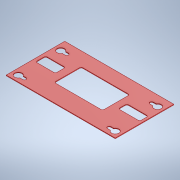
# Autodesk Inventor part: Cockpit_back_frame_cloth
Saved by Autodesk Inventor 2022 (Build 260153000, 153)
## iProperties
Part Number: Cockpit_back_frame_cloth
Material: PET プラスチック
Document SubType Name: Modeling
Designer: Masato Kubotera
Density: 1.541 g/cm^3
Appearance: 滑らか - 赤
Description: PP T0.75
Mass: 7.54732 g
Surface Area: 137.43 cm^2
Volume: 4.89767 cm^3
Author: Masato Kubotera
Autodesk Inventor part; units mm, degrees
ref_plane "YZ Plane" through (0, 0, 0) normal (1, 0, 0) x (0, 1, 0)
ref_plane "XZ Plane" through (0, 0, 0) normal (0, 1, 0) x (-1, 0, 0)
derived "Cockpit_back_frame.ipt"
sketch "スケッチ3" plane through (-88.25, 0, 0) normal (1, 0, 0) x (0, 1, 0)
  line L0 (-135, -22.5) -> (0, -22.5)
  line L1 (0, -22.5) -> (0, -39.7651)
  line L2 (0, -90) -> (-135, -90)
  line L3 (-135, -56.25) -> (0, -56.25) construction
  line L4 (-67.5, -22.5) -> (-67.5, -90) construction
  line L5 (1.4849, -41.25) -> (5, -41.25)
  line L6 (5, -41.25) -> (5, -71.25)
  line L7 (5, -71.25) -> (1.4849, -71.25)
  arc A0 (0, -39.7651) -> (1.4849, -41.25) centre (0.7425, -40.5075) ccw
  arc A1 (1.4849, -71.25) -> (0, -72.7349) centre (0.7425, -71.9925) ccw
  line L8 (0, -41.25) -> (0, -71.25)
  line L9 (0, -72.7349) -> (0, -90)
  line L10 (-135, -41.25) -> (-135, -71.25)
  line L11 (-135, -22.5) -> (-135, -39.7651)
  arc A2 (-136.4849, -41.25) -> (-135, -39.7651) centre (-135.7425, -40.5075) ccw
  line L12 (-136.4849, -41.25) -> (-140, -41.25)
  line L13 (-140, -41.25) -> (-140, -71.25)
  line L14 (-135, -72.7349) -> (-135, -90)
  arc A3 (-135, -72.7349) -> (-136.4849, -71.25) centre (-135.7425, -71.9925) ccw
  line L15 (-140, -71.25) -> (-136.4849, -71.25)
  line L16 (-100.5, -34.65) -> (-34.5, -34.65)
  line L17 (-32.5, -36.65) -> (-32.5, -66.15)
  line L18 (-34.5, -68.15) -> (-100.5, -68.15)
  line L19 (-102.5, -66.15) -> (-102.5, -36.65)
  arc A4 (-100.5, -34.65) -> (-102.5, -36.65) centre (-100.5, -36.65) ccw
  arc A5 (-102.5, -66.15) -> (-100.5, -68.15) centre (-100.5, -66.15) ccw
  arc A6 (-34.5, -68.15) -> (-32.5, -66.15) centre (-34.5, -66.15) ccw
  arc A7 (-32.5, -36.65) -> (-34.5, -34.65) centre (-34.5, -36.65) ccw
  line L20 (-126.5, -47.35) -> (-126.5, -55.45) construction
  line L21 (-118.75, -47.1) -> (-118.75, -55.7) construction
  line L22 (-110.75, -47.1) -> (-126.75, -47.1)
  line L23 (-126.75, -55.7) -> (-110.75, -47.1) construction
  line L24 (-110.75, -55.7) -> (-126.75, -47.1) construction
  line L25 (-111, -47.35) -> (-126.5, -47.35) construction
  line L26 (-111, -55.45) -> (-111, -47.35) construction
  line L27 (-111, -47.35) -> (-126.5, -55.45) construction
  circle A8 centre (-108.75, -51.4) radius 1.35
  circle A9 centre (-108.75, -51.4) radius 2.25 construction
  line L28 (-126.5, -47.35) -> (-111, -55.45) construction
  circle A10 centre (-128.75, -51.4) radius 1.35
  line L29 (-110.75, -55.7) -> (-110.75, -47.1)
  line L30 (-126.75, -55.7) -> (-110.75, -55.7)
  line L31 (-126.5, -55.45) -> (-111, -55.45) construction
  line L32 (-108.75, -51.4) -> (-128.75, -51.4) construction
  line L33 (-126.75, -47.1) -> (-126.75, -55.7)
  line L34 (-27.5, -56.65) -> (-5, -56.65) construction
  line L35 (-16.25, -46.15) -> (-16.25, -56.65) construction
  line L36 (-5, -46.15) -> (-27.5, -46.15) construction
  line L37 (-27.5, -46.15) -> (-5, -56.65) construction
  line L38 (-27.5, -56.65) -> (-5, -46.15) construction
  line L39 (-27.75, -56.9) -> (-4.75, -56.9)
  line L40 (-4.75, -45.9) -> (-27.75, -45.9)
  line L41 (-27.75, -45.9) -> (-4.75, -56.9) construction
  line L42 (-27.75, -56.9) -> (-4.75, -45.9) construction
  line L43 (-29.25, -51.4) -> (-3.25, -51.4) construction
  arc A11 (-6.2349, -56.9) -> (-4.75, -55.4151) centre (-5.4925, -56.1575) ccw
  line L44 (-5, -56.65) -> (-5, -46.15) construction
  line L45 (-4.75, -56.9) -> (-4.75, -45.9)
  arc A12 (-4.75, -47.3849) -> (-6.2349, -45.9) centre (-5.4925, -46.6425) ccw
  circle A13 centre (-3.25, -51.4) radius 0.8
  line L46 (-27.5, -46.15) -> (-27.5, -56.65) construction
  line L47 (-27.75, -45.9) -> (-27.75, -56.9)
  arc A14 (-26.2651, -45.9) -> (-27.75, -47.3849) centre (-27.0075, -46.6425) ccw
  arc A15 (-27.75, -55.4151) -> (-26.2651, -56.9) centre (-27.0075, -56.1575) ccw
  circle A16 centre (-29.25, -51.4) radius 0.8
  arc A17 (-110.75, -48.5849) -> (-112.2349, -47.1) centre (-111.4925, -47.8425) ccw
  arc A18 (-112.2349, -55.7) -> (-110.75, -54.2151) centre (-111.4925, -54.9575) ccw
  arc A19 (-126.75, -54.2151) -> (-125.2651, -55.7) centre (-126.0075, -54.9575) ccw
  arc A20 (-125.2651, -47.1) -> (-126.75, -48.5849) centre (-126.0075, -47.8425) ccw
  line L48 (-130, -29.5) -> (-130, -41.65)
  line L49 (-128, -43.65) -> (-107, -43.65)
  line L50 (-128, -27.5) -> (-126, -27.5)
  line L51 (-105, -29.5) -> (-105, -41.65)
  line L52 (-28, -27.5) -> (-21, -27.5)
  line L53 (-5, -29.5) -> (-5, -41.65)
  line L54 (-7, -43.65) -> (-28, -43.65)
  line L55 (-30, -41.65) -> (-30, -29.5)
  line L56 (-100.5, -27.5) -> (-34.5, -27.5)
  line L57 (-32.5, -29.5) -> (-32.5, -30.15)
  line L58 (-34.5, -32.15) -> (-100.5, -32.15)
  line L59 (-102.5, -30.15) -> (-102.5, -29.5)
  line L60 (-128, -59.15) -> (-107, -59.15)
  line L61 (-7, -59.15) -> (-28, -59.15)
  line L62 (-34.5, -70.65) -> (-100.5, -70.65)
  line L63 (-100.5, -85) -> (-34.5, -85)
  line L64 (-128, -85) -> (-126, -85)
  line L65 (-28, -85) -> (-21, -85)
  line L66 (-130, -61.15) -> (-130, -83)
  line L67 (-105, -61.15) -> (-105, -83)
  line L68 (-102.5, -83) -> (-102.5, -72.65)
  line L69 (-32.5, -72.65) -> (-32.5, -83)
  line L70 (-30, -83) -> (-30, -61.15)
  line L71 (-5, -61.15) -> (-5, -83)
  arc A21 (-128, -27.5) -> (-130, -29.5) centre (-128, -29.5) ccw
  arc A22 (-130, -41.65) -> (-128, -43.65) centre (-128, -41.65) ccw
  arc A23 (-107, -43.65) -> (-105, -41.65) centre (-107, -41.65) ccw
  arc A24 (-105, -29.5) -> (-107, -27.5) centre (-107, -29.5) ccw
  arc A25 (-100.5, -27.5) -> (-102.5, -29.5) centre (-100.5, -29.5) ccw
  arc A26 (-102.5, -30.15) -> (-100.5, -32.15) centre (-100.5, -30.15) ccw
  arc A27 (-34.5, -32.15) -> (-32.5, -30.15) centre (-34.5, -30.15) ccw
  arc A28 (-32.5, -29.5) -> (-34.5, -27.5) centre (-34.5, -29.5) ccw
  arc A29 (-28, -27.5) -> (-30, -29.5) centre (-28, -29.5) ccw
  arc A30 (-5, -29.5) -> (-7, -27.5) centre (-7, -29.5) ccw
  arc A31 (-7, -43.65) -> (-5, -41.65) centre (-7, -41.65) ccw
  arc A32 (-30, -41.65) -> (-28, -43.65) centre (-28, -41.65) ccw
  arc A33 (-28, -59.15) -> (-30, -61.15) centre (-28, -61.15) ccw
  arc A34 (-30, -83) -> (-28, -85) centre (-28, -83) ccw
  arc A35 (-7, -85) -> (-5, -83) centre (-7, -83) ccw
  arc A36 (-5, -61.15) -> (-7, -59.15) centre (-7, -61.15) ccw
  arc A37 (-34.5, -85) -> (-32.5, -83) centre (-34.5, -83) ccw
  arc A38 (-32.5, -72.65) -> (-34.5, -70.65) centre (-34.5, -72.65) ccw
  arc A39 (-102.5, -83) -> (-100.5, -85) centre (-100.5, -83) ccw
  arc A40 (-100.5, -70.65) -> (-102.5, -72.65) centre (-100.5, -72.65) ccw
  arc A41 (-107, -85) -> (-105, -83) centre (-107, -83) ccw
  arc A42 (-105, -61.15) -> (-107, -59.15) centre (-107, -61.15) ccw
  arc A43 (-128, -59.15) -> (-130, -61.15) centre (-128, -61.15) ccw
  arc A44 (-130, -83) -> (-128, -85) centre (-128, -83) ccw
  arc A45 (-15, -27.9) -> (-15, -32.1) centre (-15, -30) ccw construction
  circle A46 centre (-15, -30) radius 2
  circle A47 centre (-15, -30) radius 3 construction
  line L72 (-15, -32.1) -> (-11.4799, -32.1) construction
  line L73 (-15, -27.9) -> (-11.4799, -27.9) construction
  line L74 (-7.5, -30) -> (-15, -30) construction
  arc A48 (-11.4799, -32.1) -> (-11.4799, -27.9) centre (-7.5, -30) ccw construction
  arc A49 (-19, -30) -> (-11, -30) centre (-15, -30) ccw
  line L75 (-11, -30) -> (-11, -29.5)
  line L76 (-19, -30) -> (-19, -29.5)
  line L77 (-9, -27.5) -> (-7, -27.5)
  line L78 (-116, -30) -> (-116, -29.5)
  arc A50 (-124, -30) -> (-116, -30) centre (-120, -30) ccw
  circle A51 centre (-120, -30) radius 3 construction
  line L79 (-120, -32.1) -> (-123.5201, -32.1) construction
  line L80 (-120, -27.9) -> (-123.5201, -27.9) construction
  arc A52 (-120, -32.1) -> (-120, -27.9) centre (-120, -30) ccw construction
  circle A53 centre (-120, -30) radius 2
  arc A54 (-123.5201, -27.9) -> (-123.5201, -32.1) centre (-127.5, -30) ccw construction
  line L81 (-124, -30) -> (-124, -29.5)
  line L82 (-114, -27.5) -> (-107, -27.5)
  arc A55 (-123.5201, -80.4) -> (-123.5201, -84.6) centre (-127.5, -82.5) ccw construction
  line L83 (-120, -84.6) -> (-123.5201, -84.6) construction
  circle A56 centre (-120, -82.5) radius 3 construction
  circle A57 centre (-120, -82.5) radius 2
  arc A58 (-120, -84.6) -> (-120, -80.4) centre (-120, -82.5) ccw construction
  line L84 (-124, -82.5) -> (-124, -83)
  arc A59 (-116, -82.5) -> (-124, -82.5) centre (-120, -82.5) ccw
  line L85 (-116, -82.5) -> (-116, -83)
  arc A60 (-11.4799, -84.6) -> (-11.4799, -80.4) centre (-7.5, -82.5) ccw construction
  line L86 (-15, -84.6) -> (-11.4799, -84.6) construction
  circle A61 centre (-15, -82.5) radius 3 construction
  circle A62 centre (-15, -82.5) radius 2
  arc A63 (-15, -80.4) -> (-15, -84.6) centre (-15, -82.5) ccw construction
  line L87 (-15, -80.4) -> (-11.4799, -80.4) construction
  arc A64 (-11, -82.5) -> (-19, -82.5) centre (-15, -82.5) ccw
  line L88 (-19, -82.5) -> (-19, -83)
  line L89 (-7.5, -82.5) -> (-15, -82.5) construction
  line L90 (-11, -82.5) -> (-11, -83)
  line L91 (-9, -85) -> (-7, -85)
  line L92 (-120, -80.4) -> (-123.5201, -80.4) construction
  line L93 (-114, -85) -> (-107, -85)
  arc A65 (-126, -85) -> (-124, -83) centre (-126, -83) ccw
  arc A66 (-116, -83) -> (-114, -85) centre (-114, -83) ccw
  arc A67 (-124, -29.5) -> (-126, -27.5) centre (-126, -29.5) ccw
  arc A68 (-114, -27.5) -> (-116, -29.5) centre (-114, -29.5) ccw
  arc A69 (-19, -29.5) -> (-21, -27.5) centre (-21, -29.5) ccw
  arc A70 (-9, -27.5) -> (-11, -29.5) centre (-9, -29.5) ccw
  arc A71 (-21, -85) -> (-19, -83) centre (-21, -83) ccw
  arc A72 (-11, -83) -> (-9, -85) centre (-9, -83) ccw
  point P0 (0, 0)
  point P1 (-135, -71.5)
  point P2 (0, -71.5)
  point P3 (-67.5, -34.65)
  point P4 (-118.75, -51.4)
  point P5 (-118.75, -51.4)
  point P6 (-16.25, -51.4)
  point P7 (-16.25, -51.4)
  point P8 (-125, -54.6849)
  point P9 (-123.5151, -53.2)
  point P10 (-110, -60.3151)
  point P11 (-111.4849, -61.8)
  point P12 (-123.5151, -61.8)
  point P13 (-125, -60.3151)
  point P14 (-27.5151, -63)
  point P15 (-29, -61.5151)
  point P16 (-7.4849, -52)
  point P17 (-6, -53.4849)
  point P18 (-6, -61.5151)
  point P19 (-7.4849, -63)
  point P20 (-130, -27.5)
  point P21 (-130, -43.65)
  point P22 (-105, -27.5)
  point P23 (-105, -43.65)
  point P24 (-30, -27.5)
  point P25 (-5, -43.65)
  point P26 (-5, -27.5)
  point P27 (-30, -43.65)
  point P28 (-102.5, -27.5)
  point P29 (-32.5, -32.15)
  point P30 (-32.5, -27.5)
  point P31 (-102.5, -32.15)
  point P32 (-130, -59.15)
  point P33 (-105, -59.15)
  point P34 (-5, -59.15)
  point P35 (-30, -59.15)
  point P36 (-32.5, -70.65)
  point P37 (-102.5, -70.65)
  point P38 (-102.5, -85)
  point P39 (-32.5, -85)
  point P40 (-130, -85)
  point P41 (-105, -85)
  point P42 (-30, -85)
  point P43 (-5, -85)
  point P44 (-135, -71.5)
  point P45 (0, -71.5)
  point P46 (-125.5, -54.6849)
  point P47 (-124.0151, -53.2)
  point P48 (-109.5, -60.3151)
  point P49 (-110.9849, -61.8)
  point P50 (-124.0151, -61.8)
  point P51 (-125.5, -60.3151)
  point P52 (-27.5151, -63)
  point P53 (-29, -61.5151)
  point P54 (-7.4849, -52)
  point P55 (-6, -53.4849)
  point P56 (-6, -61.5151)
  point P57 (-7.4849, -63)
  point P58 (-102.5, -51.4)
  point P59 (-11, -27.5)
  point P60 (-19, -27.5)
  point P61 (-3, -30)
  point P62 (-116, -27.5)
  point P63 (-124, -27.5)
  point P64 (-124, -85)
  point P65 (-116, -85)
  point P66 (-19, -85)
  point P67 (-11, -85)
  point P68 (-118.75, -43.65)
  point P69 (-118.75, -51.4)
  point P70 (-16.25, -51.4)
ref_plane "作業平面1" through (-88.25, -135, -22.5) normal (-1, 0, 0) x (0, 1, 0)
sketch "スケッチ4" plane through (-88.25, -135, -22.5) normal (-1, 0, 0) x (0, 1, 0)
  line L0 (135, 111) -> (135, -2.5) construction
  arc A0 (102.5, 43.65) -> (100.5, 45.65) centre (100.5, 43.65) ccw projected
  line L1 (102.5, 14.15) -> (102.5, 43.65) projected
  arc A1 (100.5, 12.15) -> (102.5, 14.15) centre (100.5, 14.15) ccw projected
  line L2 (34.5, 12.15) -> (100.5, 12.15) projected
  line L3 (100.5, 45.65) -> (34.5, 45.65) projected
  line L4 (32.5, 43.65) -> (32.5, 14.15) projected
  arc A2 (32.5, 14.15) -> (34.5, 12.15) centre (34.5, 14.15) ccw projected
  arc A3 (34.5, 45.65) -> (32.5, 43.65) centre (34.5, 43.65) ccw projected
  line L5 (27.5, 34.2) -> (5, 34.2)
  line L6 (3, 32.2) -> (3, 25.6)
  line L7 (5, 23.6) -> (27.5, 23.6)
  line L8 (29.5, 25.6) -> (29.5, 32.2)
  line L9 (29.5, 34.2) -> (3, 23.6) construction
  line L10 (3, 34.2) -> (29.5, 23.6) construction
  circle A4 centre (26.25, 28.9) radius 2.25 construction
  arc A5 (29.5, 32.2) -> (27.5, 34.2) centre (27.5, 32.2) ccw
  arc A6 (5, 34.2) -> (3, 32.2) centre (5, 32.2) ccw
  arc A7 (3, 25.6) -> (5, 23.6) centre (5, 25.6) ccw
  arc A8 (27.5, 23.6) -> (29.5, 25.6) centre (27.5, 25.6) ccw
  line L11 (130, 34.15) -> (130, 23.65) construction
  line L12 (107.5, 34.15) -> (130, 34.15) construction
  line L13 (108.5, 22.65) -> (129, 22.65)
  line L14 (131, 24.65) -> (131, 33.15)
  line L15 (129, 35.15) -> (108.5, 35.15)
  line L16 (106.5, 33.15) -> (106.5, 24.65)
  line L17 (106.5, 22.65) -> (131, 35.15) construction
  line L18 (131, 22.65) -> (106.5, 35.15) construction
  arc A9 (131, 33.15) -> (129, 35.15) centre (129, 33.15) ccw
  arc A10 (108.5, 35.15) -> (106.5, 33.15) centre (108.5, 33.15) ccw
  arc A11 (106.5, 24.65) -> (108.5, 22.65) centre (108.5, 24.65) ccw
  arc A12 (129, 22.65) -> (131, 24.65) centre (129, 24.65) ccw
  line L19 (135, 67.5) -> (0, 67.5) projected
  line L20 (0, 0) -> (135, 0) projected
  line L21 (0, 0) -> (0, 67.5)
  line L22 (135, 67.5) -> (135, 0)
  line L23 (24.25, 24.6) -> (8.25, 24.6) projected
  line L24 (24.25, 33.2) -> (24.25, 24.6) projected
  line L25 (8.25, 33.2) -> (24.25, 33.2) projected
  line L26 (8.25, 24.6) -> (8.25, 33.2) projected
  arc A13 (123.5201, 5.4) -> (123.5201, 9.6) centre (127.5, 7.5) ccw projected
  line L27 (120, 5.4) -> (123.5201, 5.4) projected
  arc A14 (120, 9.6) -> (120, 5.4) centre (120, 7.5) ccw projected
  line L28 (120, 9.6) -> (123.5201, 9.6) projected
  arc A15 (123.5201, 57.9) -> (123.5201, 62.1) centre (127.5, 60) ccw projected
  line L29 (120, 62.1) -> (123.5201, 62.1) projected
  line L30 (120, 57.9) -> (123.5201, 57.9) projected
  arc A16 (120, 62.1) -> (120, 57.9) centre (120, 60) ccw projected
  line L31 (15, 9.6) -> (11.4799, 9.6) projected
  arc A17 (15, 5.4) -> (15, 9.6) centre (15, 7.5) ccw projected
  line L32 (15, 5.4) -> (11.4799, 5.4) projected
  arc A18 (11.4799, 9.6) -> (11.4799, 5.4) centre (7.5, 7.5) ccw projected
  line L33 (15, 62.1) -> (11.4799, 62.1) projected
  arc A19 (11.4799, 62.1) -> (11.4799, 57.9) centre (7.5, 60) ccw projected
  arc A20 (15, 57.9) -> (15, 62.1) centre (15, 60) ccw projected
  line L34 (15, 57.9) -> (11.4799, 57.9) projected
  line L35 (135, -5) -> (0, -5)
  line L36 (135, -5) -> (135, 0)
  line L37 (0, 0) -> (0, -5)
  line L38 (97.5, 43.65) -> (97.5, 14.15)
  line L39 (95.5, 12.15) -> (39.5, 12.15)
  line L40 (37.5, 43.65) -> (37.5, 14.15)
  line L41 (39.5, 45.65) -> (95.5, 45.65)
  arc A21 (97.5, 43.65) -> (95.5, 45.65) centre (95.5, 43.65) ccw
  arc A22 (39.5, 45.65) -> (37.5, 43.65) centre (39.5, 43.65) ccw
  arc A23 (37.5, 14.15) -> (39.5, 12.15) centre (39.5, 14.15) ccw
  arc A24 (95.5, 12.15) -> (97.5, 14.15) centre (95.5, 14.15) ccw
  line L42 (67.5, 67.5) -> (67.5, -5) construction
  point P0 (135, -22.5)
  point P1 (135, 33.75)
  point P2 (135, 24)
  point P3 (135, 24)
  point P4 (135, 24)
  point P5 (135, 44)
  point P6 (135, 44)
  point P7 (135, 44)
  point P8 (24.25, 31.7151)
  point P9 (16.25, 28.9)
  point P10 (118.75, 28.9)
  point P11 (97.5, 45.65)
  point P12 (97.5, 12.15)
  point P13 (37.5, 12.15)
  point P14 (37.5, 45.65)
  point P15 (39.5, 45.65)
  point P16 (95.5, 45.65)
  dimension "d8" = 1
  dimension "d10" = 2
  dimension "d11" = 2
  dimension "d12" = 1
  dimension "d13" = 1
  dimension "d14" = 1
  dimension "d20" = 5
  constraints: 44 end point, 28 point on line, 24 point on circle, 24 tangent, 12 centre point, 10 equal radius, 6 parallel, 5 midpoint, 4 vertical, 3 horizontal, 3 perpendicular, 2 other
  measures "d8" distance edge to line of A4 L8
  measures "d10" radius of A5
  measures "d11" radius of A9
  measures "d12" distance between parallel lines of L14 L11
  measures "d13" distance between parallel lines of L15 L12
  measures "d14" distance between parallel lines of L7 L23
  measures "d20" distance between parallel lines of L38 L1
extrude "押し出し1" add sketch "スケッチ4" along normal blind 0.75 contours L1 A1 L2 A24 L38 A21 L3 A0 | A22 L40 A23 L2 A2 L4 A3 L3 | L22 L20 L21 L19 | L36 L35 L37 L20
sketch "スケッチ2" plane through (0, 0, 0) normal (0, 1, 0) x (-1, 0, 0)
  line L0 (-23.5, -22.5) -> (-28.5, -27.5) projected
  line L1 (-28.5, -27.5) -> (-28.5, -91) projected
  line L2 (-28.5, -91) -> (-23.5, -96) projected
  line L3 (-23.5, -96) -> (34.25, -96) projected
  line L4 (36.25, -98) -> (36.25, -128.5) projected
  line L5 (36.25, -128.5) -> (46.25, -138.5) projected
  line L6 (46.25, -138.5) -> (86.5, -138.5) projected
  line L7 (91.5, -133.5) -> (91.5, -20) projected
  line L8 (91.5, -20) -> (89, -17.5) projected
  line L9 (89, -17.5) -> (83.25, -17.5) projected
  line L10 (83.25, -17.5) -> (83.25, -21.0151) projected
  line L11 (81.7651, -22.5) -> (76.8599, -22.5) projected
  line L12 (75.375, -21.0151) -> (75.375, -17.5) projected
  line L13 (75.375, -17.5) -> (60.375, -17.5) projected
  line L14 (60.375, -17.5) -> (60.375, -21.0151) projected
  line L15 (58.8901, -22.5) -> (-23.5, -22.5) projected
  line L16 (-25.25, -25) -> (-20.25, -25) construction
  line L17 (-20.25, -25) -> (-20.25, -93.5) construction
  line L18 (-20.25, -93.5) -> (-25.25, -93.5) construction
  line L19 (-25.25, -93.5) -> (-25.25, -25) construction
  line L20 (-26, -25) -> (-25.25, -25) construction
  line L21 (-25.25, -93.5) -> (-26, -93.5) construction
  line L22 (-26, -93.5) -> (-26, -25) construction
  line L23 (-20.25, -93.5) -> (83.25, -93.5) construction
  line L24 (-20.25, -88.5) -> (83.25, -88.5) construction
  line L25 (83.25, -22.5) -> (83.25, -90) construction
  line L26 (83.25, -90) -> (88.25, -90) construction
  line L27 (88.25, -90) -> (88.25, -22.5) construction
  line L28 (83.25, -88.5) -> (83.25, -93.5) construction
  line L29 (83.25, -91) -> (88.25, -91) construction
  line L30 (88.25, -91) -> (88.25, -136) construction
  line L31 (83.25, -91) -> (83.25, -136) construction
  line L32 (83.25, -136) -> (88.25, -136) construction
  line L33 (38.75, -131) -> (38.75, -93.5) construction
  line L34 (43.75, -93.5) -> (43.75, -131) construction
  line L35 (38.75, -131) -> (43.75, -131) construction
  line L36 (41.25, -131) -> (41.25, -93.5) construction
  line L37 (43.75, -131) -> (81.25, -131) construction
  line L38 (81.25, -131) -> (81.25, -136) construction
  line L39 (81.25, -136) -> (43.75, -136) construction
  line L40 (43.75, -133.5) -> (81.25, -133.5) construction
  line L41 (85.75, -91) -> (85.75, -136) construction
  circle A0 centre (85.75, -133.5) radius 2.975 projected
  arc A1 (83.25, -131) -> (88.25, -131) centre (85.75, -133.5) ccw construction
  line L42 (83.25, -91) -> (-20.25, -91) construction
  line L43 (41.25, -112.25) -> (43.75, -112.25) construction
  line L44 (62.5, -131) -> (62.5, -133.5) construction
  line L45 (41.2, -116.8151) -> (41.2, -107.6849) projected
  line L46 (43.8, -108.3) -> (43.8, -116.2) projected
  line L47 (43.8, -118.3) -> (41.2, -106.2) construction
  line L48 (41.2, -118.3) -> (43.8, -106.2) construction
  line L49 (58.55, -130.95) -> (66.45, -130.95) projected
  line L50 (67.0651, -133.55) -> (57.9349, -133.55) projected
  line L51 (56.45, -130.95) -> (68.55, -133.55) construction
  line L52 (68.55, -130.95) -> (56.45, -133.55) construction
  line L53 (41.25, -106.25) -> (43.75, -106.25) construction
  line L54 (41.25, -118.25) -> (43.75, -118.25) construction
  arc A2 (42.6849, -106.2) -> (41.2, -107.6849) centre (41.9425, -106.9425) ccw projected
  arc A3 (43.8, -108.3) -> (43.8, -106.2) centre (43.8, -107.25) ccw projected
  arc A4 (41.2, -116.8151) -> (42.6849, -118.3) centre (41.9425, -117.5575) ccw projected
  arc A5 (43.8, -118.3) -> (43.8, -116.2) centre (43.8, -117.25) ccw projected
  line L55 (56.5, -133.5) -> (56.5, -131) construction
  line L56 (68.5, -131) -> (68.5, -133.5) construction
  arc A6 (56.45, -132.0651) -> (57.9349, -133.55) centre (57.1925, -132.8075) ccw projected
  arc A7 (58.55, -130.95) -> (56.45, -130.95) centre (57.5, -130.95) ccw projected
  arc A8 (67.0651, -133.55) -> (68.55, -132.0651) centre (67.8075, -132.8075) ccw projected
  arc A9 (68.55, -130.95) -> (66.45, -130.95) centre (67.5, -130.95) ccw projected
  line L57 (56.45, -132.0651) -> (56.45, -130.95) projected
  line L58 (68.55, -130.95) -> (68.55, -132.0651) projected
  line L59 (42.6849, -106.2) -> (43.8, -106.2) projected
  line L60 (43.8, -118.3) -> (42.6849, -118.3) projected
  circle A10 centre (48.75, -133.5) radius 1.6 projected
  line L61 (88.25, -22.5) -> (88.25, -17.5) construction
  line L62 (89, -17.5) -> (89, -90) construction
  line L63 (89, -90) -> (88.25, -90) construction
  line L64 (-13.5, -82.5) -> (-13.5, -61) projected
  arc A11 (-13.5, -82.5) -> (-11.5, -84.5) centre (-11.5, -82.5) ccw projected
  line L65 (45.5, -84.5) -> (-11.5, -84.5) projected
  arc A12 (45.5, -84.5) -> (47.5, -82.5) centre (45.5, -82.5) ccw projected
  line L66 (47.5, -61) -> (47.5, -82.5) projected
  arc A13 (47.5, -61) -> (45.5, -59) centre (45.5, -61) ccw projected
  line L67 (-11.5, -59) -> (45.5, -59) projected
  arc A14 (-11.5, -59) -> (-13.5, -61) centre (-11.5, -61) ccw projected
  line L68 (31.5, -88.5) -> (31.5, -91) construction
  line L69 (85.75, -22.5) -> (85.75, -90) construction
  circle A15 centre (85.75, -31.25) radius 1.6 projected
  circle A16 centre (85.75, -31.25) radius 3 projected
  circle A17 centre (85.75, -81.25) radius 1.6 projected
  circle A18 centre (85.75, -81.25) radius 3 projected
  line L70 (88.25, -22.5) -> (83.25, -22.5) construction
  arc A19 (88.25, -91) -> (83.25, -91) centre (85.75, -133.5) ccw construction
  circle A20 centre (48.75, -133.5) radius 3 projected
  circle A21 centre (41.25, -98.5) radius 1.6 projected
  circle A22 centre (41.25, -98.5) radius 3 projected
  line L71 (10.55, -88.5) -> (10.55, -91) construction
  line L72 (52.45, -88.5) -> (52.45, -91) construction
  line L73 (51.0151, -91.05) -> (11.9849, -91.05) projected
  line L74 (10.5, -89.5651) -> (10.5, -88.45) projected
  line L75 (12.6, -88.45) -> (50.4, -88.45) projected
  line L76 (52.5, -88.45) -> (52.5, -89.5651) projected
  line L77 (52.5, -91.05) -> (10.5, -88.45) construction
  line L78 (10.5, -91.05) -> (52.5, -88.45) construction
  arc A23 (12.6, -88.45) -> (10.5, -88.45) centre (11.55, -88.45) ccw projected
  arc A24 (10.5, -89.5651) -> (11.9849, -91.05) centre (11.2425, -90.3075) ccw projected
  arc A25 (52.5, -88.45) -> (50.4, -88.45) centre (51.45, -88.45) ccw projected
  arc A26 (51.0151, -91.05) -> (52.5, -89.5651) centre (51.7575, -90.3075) ccw projected
  line L79 (-20.25, -31) -> (83.25, -31) construction
  line L80 (83.25, -26) -> (-20.25, -26) construction
  line L81 (-20.25, -26) -> (-20.25, -31) construction
  line L82 (-20.25, -28.5) -> (83.25, -28.5) construction
  line L83 (31.5, -31) -> (31.5, -26) construction
  line L84 (11.9849, -31) -> (51.0151, -31) projected
  arc A27 (10.5, -29.5151) -> (11.9849, -31) centre (11.2425, -30.2575) ccw projected
  arc A28 (51.0151, -31) -> (52.5, -29.5151) centre (51.7575, -30.2575) ccw projected
  line L85 (10.55, -31) -> (10.55, -26) construction
  line L86 (52.45, -26) -> (52.45, -31) construction
  circle A29 centre (6.5, -28.5) radius 1.6 projected
  circle A30 centre (6.5, -28.5) radius 3 projected
  line L87 (-26, -59.25) -> (-25.25, -59.25) construction
  line L88 (-22.75, -25) -> (-22.75, -93.5) construction
  arc A31 (58.8901, -22.5) -> (60.375, -21.0151) centre (59.6325, -21.7575) ccw projected
  arc A32 (75.375, -21.0151) -> (76.8599, -22.5) centre (76.1175, -21.7575) ccw projected
  line L89 (56.4375, -22.5) -> (56.4375, -17.5) construction
  line L90 (79.3125, -22.5) -> (79.3125, -17.5) construction
  circle A33 centre (-22.75, -31.75) radius 1.6 projected
  circle A34 centre (-22.75, -31.75) radius 3 projected
  circle A35 centre (-22.75, -86.75) radius 1.6 projected
  circle A36 centre (-22.75, -86.75) radius 3 projected
  line L91 (60.375, -22.5) -> (75.375, -22.5) projected
  line L92 (52.5, -17.5) -> (52.5, -22.5) construction
  circle A37 centre (85.75, -98.5) radius 1.475 projected
  circle A38 centre (85.75, -103.5) radius 1.475 projected
  circle A39 centre (85.75, -108.5) radius 1.475 projected
  line L93 (59.5, -88.5) -> (78.75, -88.5) projected
  line L94 (80.75, -90.5) -> (80.75, -126.5) projected
  line L95 (78.75, -128.5) -> (48.25, -128.5) projected
  line L96 (46.25, -126.5) -> (46.25, -110) projected
  arc A40 (46.25, -126.5) -> (48.25, -128.5) centre (48.25, -126.5) ccw projected
  arc A41 (78.75, -128.5) -> (80.75, -126.5) centre (78.75, -126.5) ccw projected
  arc A42 (80.75, -90.5) -> (78.75, -88.5) centre (78.75, -90.5) ccw projected
  arc A43 (36.25, -98) -> (34.25, -96) centre (34.25, -98) ccw projected
  circle A44 centre (-13.5, -55) radius 1.75 projected
  circle A45 centre (-13.5, -55) radius 2 projected
  line L97 (23.9, -43.85) -> (10.1, -43.85) construction
  line L98 (10.1, -43.85) -> (10.1, -34.65) construction
  line L99 (10.1, -34.65) -> (23.9, -34.65) construction
  line L100 (23.9, -34.65) -> (23.9, -43.85) construction
  line L101 (23.9, -43.85) -> (10.1, -34.65) construction
  line L102 (10.1, -43.85) -> (23.9, -34.65) construction
  line L103 (9.45, -33.95) -> (24.55, -33.95) construction
  line L104 (24.55, -33.95) -> (24.55, -44.55) construction
  line L105 (24.55, -44.55) -> (9.45, -44.55) construction
  line L106 (9.45, -44.55) -> (9.45, -33.95) construction
  line L107 (9.45, -33.95) -> (24.55, -44.55) construction
  line L108 (24.55, -33.95) -> (9.45, -44.55) construction
  line L109 (10.8849, -33.9) -> (23.1151, -33.9) projected
  line L110 (24.6, -35.3849) -> (24.6, -43.1151) projected
  line L111 (24.6, -44.6) -> (9.4, -33.9) construction
  line L112 (9.4, -44.6) -> (24.6, -33.9) construction
  line L113 (23.95, -43.9) -> (10.05, -34.6) construction
  line L114 (10.05, -43.9) -> (23.95, -34.6) construction
  arc A46 (10.8849, -33.9) -> (9.4, -35.3849) centre (10.1425, -34.6425) ccw projected
  arc A47 (11.5349, -34.6) -> (10.05, -36.0849) centre (10.7925, -35.3425) ccw projected
  line L115 (9.4, -39.25) -> (24.6, -39.25) construction
  line L116 (17, -33.9) -> (17, -44.6) construction
  arc A48 (24.6, -35.3849) -> (23.1151, -33.9) centre (23.8575, -34.6425) ccw projected
  arc A49 (23.95, -36.0849) -> (22.4651, -34.6) centre (23.2075, -35.3425) ccw projected
  arc A50 (9.4, -43.1151) -> (10.8849, -44.6) centre (10.1425, -43.8575) ccw projected
  arc A51 (10.05, -42.4151) -> (11.5349, -43.9) centre (10.7925, -43.1575) ccw projected
  arc A52 (23.1151, -44.6) -> (24.6, -43.1151) centre (23.8575, -43.8575) ccw projected
  arc A53 (22.4651, -43.9) -> (23.95, -42.4151) centre (23.2075, -43.1575) ccw projected
  line L117 (11.5349, -34.6) -> (22.4651, -34.6) projected
  line L118 (23.95, -36.0849) -> (23.95, -42.4151) projected
  line L119 (9.4, -43.1151) -> (9.4, -35.3849) projected
  line L120 (10.05, -42.4151) -> (10.05, -36.0849) projected
  line L121 (22.4651, -43.9) -> (11.5349, -43.9) projected
  line L122 (23.1151, -44.6) -> (10.8849, -44.6) projected
  line L123 (-13.5, -71.75) -> (47.5, -71.75) construction
  line L124 (85.75, -56.25) -> (88.25, -56.25) construction
  line L125 (85.7, -69.2) -> (85.7, -43.3) projected
  line L126 (88.3049, -71.3569) -> (85.7, -41.2) construction
  line L127 (85.7, -71.3) -> (88.3, -41.2) construction
  arc A54 (85.7, -41.2) -> (85.7, -43.3) centre (85.7, -42.25) ccw projected
  arc A55 (88.3, -42.6849) -> (86.8151, -41.2) centre (87.5575, -41.9425) ccw projected
  arc A56 (85.7, -69.2) -> (85.7, -71.3) centre (85.7, -70.25) ccw projected
  arc A57 (86.8151, -71.3) -> (88.3, -69.8151) centre (87.5575, -70.5575) ccw projected
  line L128 (85.75, -41.25) -> (88.25, -41.25) construction
  line L129 (85.75, -71.25) -> (88.25, -71.25) construction
  line L130 (88.25, -46.5) -> (89, -46.5) construction
  line L131 (88.25, -66.5) -> (89, -66.5) construction
  line L132 (88.3, -42.6849) -> (88.3, -69.8151) projected
  line L133 (88.3, -66.8652) -> (88.3, -69.8151) projected
  line L134 (86.8151, -71.3) -> (85.7, -71.3) projected
  line L135 (85.7, -41.2) -> (86.8151, -41.2) projected
  line L136 (86.5, -138.5) -> (91.5, -133.5) projected
  arc A58 (81.7651, -22.5) -> (83.25, -21.0151) centre (82.5075, -21.7575) ccw projected
  circle A59 centre (85.75, -93.5) radius 2 projected
  circle A60 centre (85.75, -93.5) radius 4 construction
  arc A61 (-13.5, -49) -> (-11.5, -51) centre (-11.5, -49) ccw construction
  line L137 (45.5, -51) -> (-11.5, -51) construction
  arc A62 (45.5, -51) -> (47.5, -49) centre (45.5, -49) ccw construction
  line L138 (10.5, -29.5151) -> (10.5, -22.5) projected
  line L139 (52.5, -29.5151) -> (52.5, -22.5) projected
  line L140 (67.875, -17.5) -> (67.875, -22.5) construction
  line L141 (52.5, -17.5) -> (83.25, -17.5) construction
  line L142 (43.75, -131) -> (43.75, -136) construction
  line L143 (57.5, -22.5) -> (57.5, -103) construction
  line L144 (57.5, -103) -> (52.5, -108) construction
  line L145 (-23.5, -108) -> (52.5, -108) construction
  line L146 (57.5, -90.5) -> (57.5, -103) projected
  line L147 (57.5, -103) -> (52.5, -108) projected
  line L148 (52.5, -108) -> (48.25, -108) projected
  arc A63 (59.5, -88.5) -> (57.5, -90.5) centre (59.5, -90.5) ccw projected
  arc A64 (48.25, -108) -> (46.25, -110) centre (48.25, -110) ccw projected
  circle A65 centre (56.5, -28.5) radius 1.6 projected
  circle A66 centre (56.5, -28.5) radius 3 projected
  line L149 (-13.5, -49) -> (-13.5, -29.5) projected
  point P0 (0, 0)
  point P1 (-25.7227, -96)
  point P2 (-23.5, -22.5)
  point P3 (42.5, -112.25)
  point P4 (62.5, -132.25)
  point P5 (31.5, -89.75)
  point P6 (31.5, -28.5)
  point P7 (52.5, -22)
  point P8 (46.25, -108)
  point P9 (57.5, -88.5)
  point P10 (17, -39.25)
  point P11 (17, -39.25)
  point P12 (87, -56.25)
  point P13 (17, -51)
  point P14 (10.5, -31)
  point P15 (-13.5, -39.25)
  dimension "d4" = 0.75
  constraints: 4 end point, 1 vertical
  measures "d4" distance of L62.end L26.end
equation "\"d12\" = d8"
equation "\"d13\" = d12"
equation "\"d14\" = d8"
equation "\"d2\" = d4"
